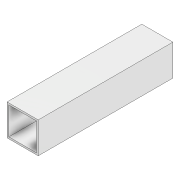
# Autodesk Inventor part: Cablecanal Ranurado 30 x 30 L = 403
Saved by Autodesk Inventor 2020 (Build 240168000, 168)
## iProperties
Created: 2020-07-02
Part Number: Cablecanal Ranurado 30 x 30 L = 403
Material: PVC-Piping
Document SubType Name: Modeling
Designer: Hernan
Density: 1.4 g/cm^3
Appearance: Smooth - White
Author: Hernan
Autodesk Inventor part; units mm, degrees
ref_plane "YZ Plane" through (0, 0, 0) normal (1, 0, 0) x (0, 1, 0)
ref_plane "XZ Plane" through (0, 0, 0) normal (0, 1, 0) x (-1, 0, 0)
ref_plane "XY Plane" through (0, 0, 0) normal (0, 0, 1) x (1, 0, 0)
sketch "Sketch1" plane through (0, 0, 0) normal (0, 0, 1) x (1, 0, 0)
  line L0 (-13.9879, -6.06) -> (16.0121, -6.06)
  line L1 (16.0121, -6.06) -> (16.0121, 23.94)
  line L2 (16.0121, 23.94) -> (-13.9879, 23.94)
  line L3 (-13.9879, 23.94) -> (-13.9879, -6.06)
  line L4 (-12.2879, 23.94) -> (-12.2879, -6.06)
  line L5 (-13.9879, -4.36) -> (16.0121, -4.36)
  line L6 (14.3121, -6.06) -> (14.3121, 23.94)
  line L7 (16.0121, 22.24) -> (-13.9879, 22.24)
  point P0 (0, 0)
  point P1 (14.3121, 22.24)
  point P2 (-12.2879, 22.24)
  point P3 (-12.2879, -4.36)
  point P4 (14.3121, -4.36)
  dimension "d1" = 30
  dimension "d3" = 1.7
  dimension "d4" = 1.7
  dimension "d5" = 1.7
  dimension "d6" = 1.7
  constraints: 16 end point, 8 point on line, 3 horizontal, 3 vertical, 2 perpendicular
  measures "d1" distance of L0.end L1.end
  measures "d3" distance between parallel lines of L2 L7
  measures "d4" distance between parallel lines of L3 L4
  measures "d5" distance between parallel lines of L1 L6
  measures "d6" distance between parallel lines of L0 L5
extrude "Extrusion1" add sketch "Sketch1" against normal blind 129.75
extrude "Extrusion2" cut sketch "Sketch1" against normal blind 403 contours L4 L7 L6 L5
body "Solid1"
